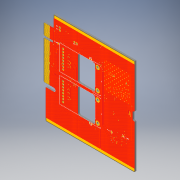
# Autodesk Inventor part: CardStandard
Saved by Autodesk Inventor 2018 (Build 220112000, 112)
## iProperties
Created: 2018-01-15
Part Number: CardStandard
Material: Epoxy Resin
Document SubType Name: Modeling
Designer: Bradley
Density: 1.14 g/cm^3
Appearance: Smooth - Medium Gray
Mass: 15.4834 g
Surface Area: 175.95 cm^2
Volume: 13.582 cm^3
Author: Bradley
Revision Number: 3.1
Autodesk Inventor part; units mm, degrees
ref_plane "YZ Plane" through (0, 0, 0) normal (1, 0, 0) x (0, 1, 0)
ref_plane "XZ Plane" through (0, 0, 0) normal (0, 1, 0) x (-1, 0, 0)
ref_plane "XY Plane" through (0, 0, 0) normal (0, 0, 1) x (1, 0, 0)
sketch "Sketch1" plane through (0, 0, 0) normal (0, 0, 1) x (1, 0, 0)
  line L0 (0, 36.15) -> (10, 36.15)
  line L1 (10, 36.15) -> (10, 47.9)
  line L2 (10, 47.9) -> (90.4, 47.9)
  line L3 (90.4, 47.9) -> (90.4, -47.9)
  line L4 (90.4, -47.9) -> (2, -47.9)
  line L5 (10, -15.15) -> (0, -15.15)
  line L6 (-5.5, 48) -> (90.5, 48) construction
  line L7 (90.5, 48) -> (90.5, -48) construction
  line L8 (90.5, -48) -> (-5.5, -48) construction
  line L9 (-5.5, -48) -> (-5.5, 48) construction
  line L10 (-5.4, 47.9) -> (-3.4, 47.9) construction
  line L11 (-3.4, 47.9) -> (-3.4, -47.9) construction
  line L12 (-3.4, -47.9) -> (-5.4, -47.9) construction
  line L13 (-5.4, -47.9) -> (-5.4, 47.9) construction
  line L14 (-3.4, 38.5) -> (7.85, 38.5) construction
  line L15 (7.85, 38.5) -> (7.85, -17.5) construction
  line L16 (7.85, -17.5) -> (-3.4, -17.5) construction
  line L17 (-3.4, -17.5) -> (-3.4, 38.5) construction
  line L18 (2, -47.9) -> (2, -18.65)
  line L19 (2, -18.65) -> (10, -18.65)
  arc A0 (10, -18.65) -> (10, -15.15) centre (10, -16.9) ccw
  line L20 (0, 24) -> (90.5, 24) construction
  circle A1 centre (-2.5, 47.1) radius 0.9 construction
  circle A2 centre (-0.7, 47.1) radius 0.9 construction
  circle A3 centre (1.1, 47.1) radius 0.9 construction
  circle A4 centre (2.9, 47.1) radius 0.9 construction
  circle A5 centre (4.7, 47.1) radius 0.9 construction
  circle A6 centre (6.5, 47.1) radius 0.9 construction
  circle A7 centre (8.3, 47.1) radius 0.9 construction
  circle A8 centre (-2.5, 45.3) radius 0.9 construction
  circle A9 centre (-0.7, 45.3) radius 0.9 construction
  circle A10 centre (1.1, 45.3) radius 0.9 construction
  circle A11 centre (2.9, 45.3) radius 0.9 construction
  circle A12 centre (4.7, 45.3) radius 0.9 construction
  circle A13 centre (6.5, 45.3) radius 0.9 construction
  circle A14 centre (8.3, 45.3) radius 0.9 construction
  circle A15 centre (-2.5, 43.5) radius 0.9 construction
  circle A16 centre (-0.7, 43.5) radius 0.9 construction
  circle A17 centre (1.1, 43.5) radius 0.9 construction
  circle A18 centre (2.9, 43.5) radius 0.9 construction
  circle A19 centre (4.7, 43.5) radius 0.9 construction
  circle A20 centre (6.5, 43.5) radius 0.9 construction
  circle A21 centre (8.3, 43.5) radius 0.9 construction
  circle A22 centre (-2.5, 41.7) radius 0.9 construction
  circle A23 centre (-0.7, 41.7) radius 0.9 construction
  circle A24 centre (1.1, 41.7) radius 0.9 construction
  circle A25 centre (2.9, 41.7) radius 0.9 construction
  circle A26 centre (4.7, 41.7) radius 0.9 construction
  circle A27 centre (6.5, 41.7) radius 0.9 construction
  circle A28 centre (8.3, 41.7) radius 0.9 construction
  circle A29 centre (-2.5, 39.9) radius 0.9 construction
  circle A30 centre (-0.7, 39.9) radius 0.9 construction
  circle A31 centre (1.1, 39.9) radius 0.9 construction
  circle A32 centre (2.9, 39.9) radius 0.9 construction
  circle A33 centre (4.7, 39.9) radius 0.9 construction
  circle A34 centre (6.5, 39.9) radius 0.9 construction
  circle A35 centre (8.3, 39.9) radius 0.9 construction
  line L21 (0, 36.15) -> (0, 24.95)
  line L22 (0, 24.95) -> (8.4, 24.95)
  arc A36 (8.4, 23.05) -> (8.4, 24.95) centre (8.4, 24) ccw
  line L23 (8.4, 23.05) -> (0, 23.05)
  line L24 (0, 23.05) -> (0, -15.15)
  point P0 (0, 0)
  point P1 (-5.5, 0)
  point P2 (90.4, 0)
  point P3 (90.5, 0)
  dimension "d0" = 51.3
  dimension "d1" = 95.8
  dimension "d3" = 10
  dimension "d20" = 96
  dimension "d21" = 96
  dimension "d22" = 0.1
  dimension "d23" = 0.1
  dimension "d24" = 2
  dimension "d25" = 0.1
  dimension "d28" = 11.25
  dimension "d29" = 56
  dimension "d31" = 9.5
  dimension "d32" = 30.5
  dimension "d34" = 3.5
  dimension "d35" = 12.15
  dimension "d36" = 39.15
  dimension "d37" = 14.5
  dimension "d38" = 1.15
  dimension "d39" = 1.8
  dimension "d42" = 1.8
  dimension "d45" = 1.8
  dimension "d48" = 2
  dimension "d49" = 3.4
  dimension "d50" = 1.9
  dimension "d51" = 8.4
  dimension "d52" = 24
  constraints: 50 end point, 37 centre point, 11 perpendicular, 7 parallel, 6 point on line, 6 tangent, 5 horizontal, 4 point on circle, 3 midpoint, 3 vertical, 2 collinear, 2 horizontal alignment, 68 other
  measures "d0" distance of L5.end L0.start
  measures "d1" distance of L2.end L3.end
  measures "d3" distance of L0.start L0.end
  measures "d20" distance of L6.start L6.end
  measures "d21" distance of L8.end L6.start
  measures "d22" distance between parallel lines of L2 L6
  measures "d23" distance between parallel lines of L7 L3
  measures "d24" distance between parallel lines of L13 L11
  measures "d25" distance between parallel lines of L13 L9
  measures "d28" distance of L15.end L16.end
  measures "d29" distance of L14.end L15.end
  measures "d31" distance between parallel lines of L14 L6
  measures "d32" distance between parallel lines of L8 L16
  measures "d34" distance between parallel lines of L5 L19
  measures "d35" distance between parallel lines of L20 L0
  measures "d36" distance between parallel lines of L5 L20
  measures "d37" distance between parallel lines of L20 L14
  measures "d38" distance between parallel lines of L19 L16
  measures "d39" diameter of A1
  measures "d42" distance of A1.centre A2.centre
  measures "d45" distance of A1.centre A8.centre
  measures "d48" distance between parallel lines of L18 L24
  measures "d49" distance between parallel lines of L24 L11
  measures "d50" distance between parallel lines of L23 L22
  measures "d51" distance of L21.end L22.end
  measures "d52" distance from line of point (0, 0) L20
extrude "Extrusion1" add sketch "Sketch1" along normal mid plane 1.6
chamfer "Chamfer1" distance 0.5 angle 45 4 edges at (0, 36.15, 0) (0, 24.95, 0) (0, 23.05, 0) (0, -15.15, 0)
fillet "Fillet1" radius 0.5 6 edges at (10, 36.15, 0) (10, 47.9, 0) (90.4, 47.9, 0) (90.4, -47.9, 0) (2, -47.9, 0) (2, -18.65, 0)
sketch "Sketch16" plane through (0, 0, 0.8) normal (0, 0, 1) x (1, 0, 0)
  arc A0 (2.5, -18.65) -> (2, -19.15) centre (2.5, -19.15) ccw projected
  line L0 (2, -19.15) -> (2, -47.4) projected
  arc A1 (2, -47.4) -> (2.5, -47.9) centre (2.5, -47.4) ccw projected
  line L1 (2.5, -47.9) -> (89.9, -47.9) projected
  arc A2 (89.9, -47.9) -> (90.4, -47.4) centre (89.9, -47.4) ccw projected
  line L2 (90.4, -47.4) -> (90.4, 47.4) projected
  arc A3 (90.4, 47.4) -> (89.9, 47.9) centre (89.9, 47.4) ccw projected
  line L3 (89.9, 47.9) -> (10.5, 47.9) projected
  arc A4 (10.5, 47.9) -> (10, 47.4) centre (10.5, 47.4) ccw projected
  line L4 (10, 47.4) -> (10, 36.65) projected
  arc A5 (9.5, 36.15) -> (10, 36.65) centre (9.5, 36.65) ccw projected
  line L5 (9.5, 36.15) -> (0.5, 36.15) projected
  line L6 (0, 35.65) -> (0.5, 36.15) projected
  line L7 (0, 35.65) -> (0, 25.45) projected
  line L8 (0.5, 24.95) -> (0, 25.45) projected
  line L9 (0.5, 24.95) -> (8.4, 24.95) projected
  arc A6 (8.4, 23.05) -> (8.4, 24.95) centre (8.4, 24) ccw projected
  line L10 (8.4, 23.05) -> (0.5, 23.05) projected
  line L11 (0, 22.55) -> (0.5, 23.05) projected
  line L12 (0, 22.55) -> (0, -14.65) projected
  line L13 (0.5, -15.15) -> (0, -14.65) projected
  line L14 (0.5, -15.15) -> (10, -15.15) projected
  arc A7 (10, -18.65) -> (10, -15.15) centre (10, -16.9) ccw projected
  line L15 (10, -18.65) -> (2.5, -18.65) projected
  line L16 (36.05, 26.5) -> (49.05, 26.5)
  line L17 (51.05, 24.5) -> (51.05, 3.5)
  line L18 (49.05, 1.5) -> (36.05, 1.5)
  line L19 (34.05, 3.5) -> (34.05, 24.5)
  line L20 (36.05, -1.5) -> (49.05, -1.5)
  line L21 (51.05, -3.5) -> (51.05, -24.5)
  line L22 (49.05, -26.5) -> (36.05, -26.5)
  line L23 (34.05, -24.5) -> (34.05, -3.5)
  line L24 (88.4, 3) -> (88.4, -3)
  arc A8 (88.4, -3) -> (89.4, -4) centre (89.4, -3) ccw
  arc A9 (90.4, -5) -> (89.4, -4) centre (89.4, -5) ccw
  arc A10 (89.4, 4) -> (88.4, 3) centre (89.4, 3) ccw
  line L25 (90.4, -47.4) -> (90.4, 47.4) projected
  arc A11 (89.4, 4) -> (90.4, 5) centre (89.4, 5) ccw
  arc A12 (36.05, 26.5) -> (34.05, 24.5) centre (36.05, 24.5) ccw
  arc A13 (51.05, 24.5) -> (49.05, 26.5) centre (49.05, 24.5) ccw
  arc A14 (49.05, 1.5) -> (51.05, 3.5) centre (49.05, 3.5) ccw
  arc A15 (51.05, -3.5) -> (49.05, -1.5) centre (49.05, -3.5) ccw
  arc A16 (49.05, -26.5) -> (51.05, -24.5) centre (49.05, -24.5) ccw
  arc A17 (34.05, -24.5) -> (36.05, -26.5) centre (36.05, -24.5) ccw
  arc A18 (36.05, -1.5) -> (34.05, -3.5) centre (36.05, -3.5) ccw
  arc A19 (34.05, 3.5) -> (36.05, 1.5) centre (36.05, 3.5) ccw
  point P0 (0, 0)
  point P1 (34.05, -1.5)
  point P2 (51.05, -26.5)
  point P3 (88.4, 0)
  dimension "d145" = 6
  dimension "d146" = 1
  dimension "d147" = 3
  dimension "d148" = 1.5
  dimension "d149" = 34.05
  dimension "d150" = 51.05
  dimension "d151" = 26.5
  dimension "d152" = 2
  constraints: 24 point on circle, 22 tangent, 18 end point, 12 centre point, 10 equal radius, 8 point on line, 4 parallel, 2 horizontal, 2 perpendicular, 1 collinear, 1 horizontal alignment, 1 midpoint, 1 vertical, 1 vertical alignment
  measures "d145" distance of L24.start L24.end
  measures "d146" radius of A11
  measures "d147" distance between parallel lines of L20 L18
  measures "d148" distance from line of point (0, 0) L18
  measures "d149" distance between parallel lines of L19 L12
  measures "d150" distance between parallel lines of L12 L17
  measures "d151" distance from line of point (0, 0) L22
  measures "d152" radius of A12
extrude "Extrusion6" cut sketch "Sketch16" against normal through all contours A9 A8 L24 A10 A11 L2 | L16 A13 L17 A14 L18 A19 L19 A12 | L20 A15 L21 A16 L22 A17 L23 A18
sketch "Sketch19" plane through (0, 0, 0.8) normal (0, 0, 1) x (1, 0, 0)
  line L0 (0, 22.55) -> (0, -14.65) projected
  line L1 (90.4, 5) -> (90.4, 47.4) projected
  line L2 (0, 47.8927) -> (90.4, 47.8927) construction
  line L3 (90.4, 47.8927) -> (90.4, -47.8927) construction
  line L4 (90.4, -47.8927) -> (0, -47.8927) construction
  line L5 (0, -47.8927) -> (0, 47.8927) construction
  point P0 (0, 0)
  constraints: 2 collinear, 1 midpoint, 2 other
decal "Decal4"
sketch "Sketch20" plane through (0, 0, -0.8) normal (0, 0, -1) x (-1, 0, 0)
  line L0 (-90.4, 47.4) -> (-90.4, 5) projected
  line L1 (0, -14.65) -> (0, 22.55) projected
  line L2 (-90.4, 47.8927) -> (0, 47.8927) construction
  line L3 (0, 47.8927) -> (0, -47.8927) construction
  line L4 (0, -47.8927) -> (-90.4, -47.8927) construction
  line L5 (-90.4, -47.8927) -> (-90.4, 47.8927) construction
  point P0 (0, 0)
  constraints: 2 collinear, 1 midpoint, 2 other
decal "Decal5"
sketch "Sketch21" plane through (0, 0, 0.8) normal (0, 0, 1) x (1, 0, 0)
  point P0 (0, 0)
  point P1 (53.55, -24)
  point P2 (53.55, -4)
  point P3 (53.55, 24)
  point P4 (53.55, 4)
  constraints: 4 other
hole "Hole9" at (53.55, -24, 0.8) at (53.55, -4, 0.8) at (53.55, 24, 0.8) at (53.55, 4, 0.8) direction (0, 0, -1) diameter 2.2 end through all
sketch "Sketch22" plane through (0, 0, 0.8) normal (0, 0, 1) x (1, 0, 0)
  point P0 (0, 0)
  point P1 (19.25, -17.81)
  point P2 (32.9, 34.25)
  point P3 (19.25, -12.73)
  point P4 (19.25, -10.19)
  point P5 (19.25, -7.65)
  point P6 (19.25, -5.11)
  point P7 (19.25, -15.27)
  point P8 (19.25, 20.35)
  point P9 (19.25, -20.35)
  point P10 (19.25, -22.89)
  point P11 (19.25, 17.81)
  point P12 (19.25, 15.27)
  point P13 (19.25, 22.89)
  point P14 (19.25, 12.73)
  point P15 (19.25, 10.19)
  point P16 (19.25, 7.65)
  point P17 (19.25, 5.11)
  point P18 (30.5, 34.25)
  point P19 (16, 39.5)
  point P20 (16, 37.05)
  constraints: 20 other
hole "Hole10" at (19.25, -17.81, 0.8) at (32.9, 34.25, 0.8) at (19.25, -12.73, 0.8) at (19.25, -10.19, 0.8) at (19.25, -7.65, 0.8) at (19.25, -5.11, 0.8) at (19.25, -15.27, 0.8) at (19.25, 20.35, 0.8) at (19.25, -20.35, 0.8) at (19.25, -22.89, 0.8) at (19.25, 17.81, 0.8) at (19.25, 15.27, 0.8) at (19.25, 22.89, 0.8) at (19.25, 12.73, 0.8) at (19.25, 10.19, 0.8) at (19.25, 7.65, 0.8) at (19.25, 5.11, 0.8) at (30.5, 34.25, 0.8) at (16, 39.5, 0.8) at (16, 37.05, 0.8) direction (0, 0, -1) diameter 1 end through all
sketch "Sketch23" plane through (0, 0, 0.8) normal (0, 0, 1) x (1, 0, 0)
  point P0 (0, 0)
  point P1 (82, 24.5)
  point P2 (69.5, 24.5)
  constraints: 2 other
hole "Hole11" at (82, 24.5, 0.8) at (69.5, 24.5, 0.8) direction (0, 0, -1) diameter 0.6 end through all
sketch "Sketch24" plane through (0, 0, 0.8) normal (0, 0, 1) x (1, 0, 0)
  point P0 (0, 0)
  point P1 (52.419, -22.869)
  point P2 (51.95, -24)
  point P3 (52.419, -25.131)
  point P4 (55.15, -24)
  point P5 (53.55, -5.6)
  point P6 (54.681, -5.131)
  point P7 (55.15, -4)
  point P8 (54.681, -2.869)
  point P9 (53.55, -2.4)
  point P10 (52.419, -2.869)
  point P11 (54.681, -22.869)
  point P12 (53.55, 22.4)
  point P13 (54.681, 22.869)
  point P14 (55.15, 24)
  point P15 (54.681, 25.131)
  point P16 (53.55, 25.6)
  point P17 (52.419, 25.131)
  point P18 (51.95, -4)
  point P19 (52.419, 22.869)
  point P20 (53.55, 2.4)
  point P21 (54.681, 2.869)
  point P22 (55.15, 4)
  point P23 (54.681, 5.131)
  point P24 (53.55, 5.6)
  point P25 (51.95, 24)
  point P26 (51.95, 4)
  point P27 (52.419, 2.869)
  point P28 (52.419, -5.131)
  point P29 (53.55, -25.6)
  point P30 (54.681, -25.131)
  point P31 (53.55, -22.4)
  point P32 (52.419, 5.131)
  constraints: 32 other
hole "Hole12" at (52.419, -22.869, 0.8) at (51.95, -24, 0.8) at (52.419, -25.131, 0.8) at (55.15, -24, 0.8) at (53.55, -5.6, 0.8) at (54.681, -5.131, 0.8) at (55.15, -4, 0.8) at (54.681, -2.869, 0.8) at (53.55, -2.4, 0.8) at (52.419, -2.869, 0.8) at (54.681, -22.869, 0.8) at (53.55, 22.4, 0.8) at (54.681, 22.869, 0.8) at (55.15, 24, 0.8) at (54.681, 25.131, 0.8) at (53.55, 25.6, 0.8) at (52.419, 25.131, 0.8) at (51.95, -4, 0.8) at (52.419, 22.869, 0.8) at (53.55, 2.4, 0.8) at (54.681, 2.869, 0.8) at (55.15, 4, 0.8) at (54.681, 5.131, 0.8) at (53.55, 5.6, 0.8) at (51.95, 24, 0.8) at (51.95, 4, 0.8) at (52.419, 2.869, 0.8) at (52.419, -5.131, 0.8) at (53.55, -25.6, 0.8) at (54.681, -25.131, 0.8) at (53.55, -22.4, 0.8) at (52.419, 5.131, 0.8) direction (0, 0, -1) diameter 0.35 end through all
sketch "Sketch25" plane through (0, 0, 0.8) normal (0, 0, 1) x (1, 0, 0)
  point P0 (0, 0)
  point P1 (80.65, 14.55)
  point P2 (79.45, 14.55)
  point P3 (79.15, 12.8)
  point P4 (79.1, 11.55)
  point P5 (77.3, 14.15)
  point P6 (76.1, 14.15)
  point P7 (77.25, 12.15)
  point P8 (77.25, 10.95)
  point P9 (74.55, 13)
  point P10 (72.7, 14.55)
  point P11 (69.6, 14.35)
  point P12 (69.8, 13)
  point P13 (69.8, 11.1)
  point P14 (72.3, 11.4)
  point P15 (66.9, 23.8)
  point P16 (68.5, 23.8)
  point P17 (64.9, 24.9)
  point P18 (68.5, 25.1)
  point P19 (66.9, 25.1)
  point P20 (64.9, 23.6)
  point P21 (82.7, 23.6)
  point P22 (81.3, 23.6)
  point P23 (82, 25.6)
  point P24 (82.7, 19.4)
  point P25 (81.3, 18.8)
  point P26 (83.8, 16.4)
  point P27 (85, 17)
  point P28 (85.05, 14.2)
  point P29 (81.1, 16.2)
  point P30 (77.95, 16.35)
  point P31 (75.05, 16.35)
  point P32 (71.85, 15.55)
  point P33 (66.5, 13.7)
  point P34 (65.6, 12.3)
  point P35 (70.6, 24.5)
  point P36 (84.5, 32)
  point P37 (76.5, 32)
  point P38 (68.5, 32)
  point P39 (72.5, 32)
  point P40 (80.5, 32)
  point P41 (64.5, 32)
  point P42 (82.5, 30)
  point P43 (74.5, 30)
  point P44 (66.5, 30)
  point P45 (70.5, 30)
  point P46 (78.5, 30)
  point P47 (62.5, 30)
  point P48 (84.5, 28)
  point P49 (76.5, 28)
  point P50 (68.5, 28)
  point P51 (72.5, 28)
  point P52 (80.5, 28)
  point P53 (64.5, 28)
  point P54 (74.5, 26)
  point P55 (66.5, 26)
  point P56 (70.5, 26)
  point P57 (78.5, 26)
  point P58 (62.5, 26)
  point P59 (84.5, 24)
  point P60 (76.5, 24)
  point P61 (72.5, 24)
  point P62 (74.5, 22)
  point P63 (66.5, 22)
  point P64 (70.5, 22)
  point P65 (78.5, 22)
  point P66 (62.5, 22)
  point P67 (84.5, 20)
  point P68 (76.5, 20)
  point P69 (68.5, 20)
  point P70 (72.5, 20)
  point P71 (80.5, 20)
  point P72 (64.5, 20)
  point P73 (74.5, 18)
  point P74 (66.5, 18)
  point P75 (70.5, 18)
  point P76 (78.5, 18)
  point P77 (62.5, 18)
  point P78 (84.5, 8)
  point P79 (76.5, 8)
  point P80 (68.5, 8)
  point P81 (72.5, 8)
  point P82 (80.5, 8)
  point P83 (64.5, 8)
  point P84 (82.5, 10)
  point P85 (74.5, 10)
  point P86 (66.5, 10)
  point P87 (70.5, 10)
  point P88 (78.5, 10)
  point P89 (62.5, 10)
  point P90 (82.5, 34)
  point P91 (74.5, 34)
  point P92 (66.5, 34)
  point P93 (70.5, 34)
  point P94 (56.2, 27.1)
  point P95 (62.5, 34)
  point P96 (60.5, 32)
  point P97 (60.5, 28)
  point P98 (60.5, 24)
  point P99 (60.5, 20)
  point P100 (60.5, 16)
  point P101 (62.5, 14)
  point P102 (60.5, 12)
  point P103 (64.5, 12)
  point P104 (64.5, 16)
  point P105 (13.5, 24.2)
  point P106 (15.3, 2.5)
  point P107 (15.3, -4.8)
  point P108 (55.3, -27)
  point P109 (73.075, -22.125)
  point P110 (77.7, -26.1)
  point P111 (25, 9.9)
  point P112 (25, 12.8)
  point P113 (25, 15.9)
  point P114 (24.59, 18.9)
  point P115 (24.6, -9.1)
  point P116 (25, -18.1)
  point P117 (25, -15.1)
  point P118 (25, -12.1)
  point P119 (80.4, -20.2)
  point P120 (80.4, -17.9)
  point P121 (62.6, 1.8)
  point P122 (60.2, 3.5)
  point P123 (25.25, 1.4)
  point P124 (25.25, -1.4)
  point P125 (28.5, 1.4)
  point P126 (13.8, 20)
  point P127 (67.5, -26.2)
  point P128 (58.86, 23)
  point P129 (67, -31)
  point P130 (72.9, -30.3)
  point P131 (69.3, -28.5)
  point P132 (67, -28.5)
  point P133 (55.5, 29.3)
  point P134 (57.7, 27.5)
  point P135 (57.7, 25.6)
  point P136 (72.5, -32.1)
  point P137 (87.6, 7.7)
  point P138 (70.3, -30.7)
  point P139 (68.7, -33.25)
  point P140 (70.432, -27.94)
  point P141 (77.1, -30.9)
  point P142 (72.3, -26.4)
  point P143 (58.3, 24.9)
  point P144 (67, -32.3)
  point P145 (72.4, -30.9)
  point P146 (69.3, -29.8)
  point P147 (51.75, -29.75)
  point P148 (70.001, -7.599)
  point P149 (69.209, -8.391)
  point P150 (77.45, -23.85)
  point P151 (6, -2.5)
  point P152 (30.5, -2.4)
  point P153 (26.4, 14.45)
  point P154 (6, -3.5)
  point P155 (31.1, -3)
  point P156 (29.9, -3)
  point P157 (29.9, -1.8)
  point P158 (26.4, 13.6)
  point P159 (6, -4.5)
  point P160 (31.7, -3.6)
  point P161 (29.3, -3.6)
  point P162 (29.3, -1.2)
  point P163 (26.4, 11.45)
  point P164 (58, 30.4)
  point P165 (17.6, 8.9)
  point P166 (26.4, 10.1)
  point P167 (9.8, 5.2)
  point P168 (20.7, -1.4)
  point P169 (24.5, -5.2)
  point P170 (6, 34.5)
  point P171 (6, 4.5)
  point P172 (6, 3.5)
  point P173 (27.596, 0.396)
  point P174 (26.804, -0.396)
  point P175 (25.3, 18.4)
  point P176 (25.8, 15.4)
  point P177 (25.8, 12.4)
  point P178 (25.3, -9.6)
  point P179 (25.8, -12.6)
  point P180 (25.8, -15.6)
  point P181 (6, 35.5)
  point P182 (25.2, 21)
  point P183 (26.4, -5.9)
  point P184 (32.4, -0.76)
  point P185 (70.6, 4.6)
  point P186 (70.75, 6.25)
  point P187 (6, 33.5)
  point P188 (6, 32.5)
  point P189 (6, 31.5)
  point P190 (6, 30.5)
  point P191 (6, 29.5)
  point P192 (6, 28.5)
  point P193 (6, 27.5)
  point P194 (6, 26.5)
  point P195 (6, 20.5)
  point P196 (6, 19.5)
  point P197 (6, 18.5)
  point P198 (6, 17.5)
  point P199 (6, 16.5)
  constraints: 244 other
hole "Hole13" at (80.65, 14.55, 0.8) at (79.45, 14.55, 0.8) at (79.15, 12.8, 0.8) at (79.1, 11.55, 0.8) at (77.3, 14.15, 0.8) at (76.1, 14.15, 0.8) at (77.25, 12.15, 0.8) at (77.25, 10.95, 0.8) at (74.55, 13, 0.8) at (72.7, 14.55, 0.8) at (69.6, 14.35, 0.8) at (69.8, 13, 0.8) at (69.8, 11.1, 0.8) at (72.3, 11.4, 0.8) at (66.9, 23.8, 0.8) at (68.5, 23.8, 0.8) at (64.9, 24.9, 0.8) at (68.5, 25.1, 0.8) at (66.9, 25.1, 0.8) at (64.9, 23.6, 0.8) at (82.7, 23.6, 0.8) at (81.3, 23.6, 0.8) at (82, 25.6, 0.8) at (82.7, 19.4, 0.8) at (81.3, 18.8, 0.8) at (83.8, 16.4, 0.8) at (85, 17, 0.8) at (85.05, 14.2, 0.8) at (81.1, 16.2, 0.8) at (77.95, 16.35, 0.8) at (75.05, 16.35, 0.8) at (71.85, 15.55, 0.8) at (66.5, 13.7, 0.8) at (65.6, 12.3, 0.8) at (70.6, 24.5, 0.8) at (84.5, 32, 0.8) at (76.5, 32, 0.8) at (68.5, 32, 0.8) at (72.5, 32, 0.8) at (80.5, 32, 0.8) at (64.5, 32, 0.8) at (82.5, 30, 0.8) at (74.5, 30, 0.8) at (66.5, 30, 0.8) at (70.5, 30, 0.8) at (78.5, 30, 0.8) at (62.5, 30, 0.8) at (84.5, 28, 0.8) at (76.5, 28, 0.8) at (68.5, 28, 0.8) direction (0, 0, -1) diameter 0.3 end through all and at (72.5, 28, 0.8) (80.5, 28, 0.8) (64.5, 28, 0.8) (74.5, 26, 0.8) (66.5, 26, 0.8) (70.5, 26, 0.8) (78.5, 26, 0.8) (62.5, 26, 0.8) (84.5, 24, 0.8) (76.5, 24, 0.8) (72.5, 24, 0.8) (74.5, 22, 0.8) (66.5, 22, 0.8) (70.5, 22, 0.8) (78.5, 22, 0.8) (62.5, 22, 0.8) (84.5, 20, 0.8) (76.5, 20, 0.8) (68.5, 20, 0.8) (72.5, 20, 0.8) (80.5, 20, 0.8) (64.5, 20, 0.8) (74.5, 18, 0.8) (66.5, 18, 0.8) (70.5, 18, 0.8) (78.5, 18, 0.8) (62.5, 18, 0.8) (84.5, 8, 0.8) (76.5, 8, 0.8) (68.5, 8, 0.8) (72.5, 8, 0.8) (80.5, 8, 0.8) (64.5, 8, 0.8) (82.5, 10, 0.8) (74.5, 10, 0.8) (66.5, 10, 0.8) (70.5, 10, 0.8) (78.5, 10, 0.8) (62.5, 10, 0.8) (82.5, 34, 0.8) (74.5, 34, 0.8) (66.5, 34, 0.8) (70.5, 34, 0.8) (56.2, 27.1, 0.8) (62.5, 34, 0.8) (60.5, 32, 0.8) (60.5, 28, 0.8) (60.5, 24, 0.8) (60.5, 20, 0.8) (60.5, 16, 0.8) (62.5, 14, 0.8) (60.5, 12, 0.8) (64.5, 12, 0.8) (64.5, 16, 0.8) (13.5, 24.2, 0.8) (15.3, 2.5, 0.8) (15.3, -4.8, 0.8) (55.3, -27, 0.8) (73.075, -22.125, 0.8) (77.7, -26.1, 0.8) (25, 9.9, 0.8) (25, 12.8, 0.8) (25, 15.9, 0.8) (24.59, 18.9, 0.8) (24.6, -9.1, 0.8) (25, -18.1, 0.8) (25, -15.1, 0.8) (25, -12.1, 0.8) (80.4, -20.2, 0.8) (80.4, -17.9, 0.8) (62.6, 1.8, 0.8) (60.2, 3.5, 0.8) (25.25, 1.4, 0.8) (25.25, -1.4, 0.8) (28.5, 1.4, 0.8) (13.8, 20, 0.8) (67.5, -26.2, 0.8) (58.86, 23, 0.8) (67, -31, 0.8) (72.9, -30.3, 0.8) (69.3, -28.5, 0.8) (67, -28.5, 0.8) (55.5, 29.3, 0.8) (57.7, 27.5, 0.8) (57.7, 25.6, 0.8) (72.5, -32.1, 0.8) (87.6, 7.7, 0.8) (70.3, -30.7, 0.8) (68.7, -33.25, 0.8) (70.432, -27.94, 0.8) (77.1, -30.9, 0.8) (72.3, -26.4, 0.8) (58.3, 24.9, 0.8) (67, -32.3, 0.8) (72.4, -30.9, 0.8) (69.3, -29.8, 0.8) (51.75, -29.75, 0.8) (70.001, -7.599, 0.8) (69.209, -8.391, 0.8) (77.45, -23.85, 0.8) (6, -2.5, 0.8) (30.5, -2.4, 0.8) (26.4, 14.45, 0.8) (6, -3.5, 0.8) (31.1, -3, 0.8) (29.9, -3, 0.8) (29.9, -1.8, 0.8) (26.4, 13.6, 0.8) (6, -4.5, 0.8) (31.7, -3.6, 0.8) (29.3, -3.6, 0.8) (29.3, -1.2, 0.8) (26.4, 11.45, 0.8) (58, 30.4, 0.8) (17.6, 8.9, 0.8) (26.4, 10.1, 0.8) (9.8, 5.2, 0.8) (20.7, -1.4, 0.8) (24.5, -5.2, 0.8) (6, 34.5, 0.8) (6, 4.5, 0.8) (6, 3.5, 0.8) (27.596, 0.396, 0.8) (26.804, -0.396, 0.8) (25.3, 18.4, 0.8) (25.8, 15.4, 0.8) (25.8, 12.4, 0.8) (25.3, -9.6, 0.8) (25.8, -12.6, 0.8) (25.8, -15.6, 0.8) (6, 35.5, 0.8) (25.2, 21, 0.8) (26.4, -5.9, 0.8) (32.4, -0.76, 0.8) (70.6, 4.6, 0.8) (70.75, 6.25, 0.8) (6, 33.5, 0.8) (6, 32.5, 0.8) (6, 31.5, 0.8) (6, 30.5, 0.8) (6, 29.5, 0.8) (6, 28.5, 0.8) (6, 27.5, 0.8) (6, 26.5, 0.8) (6, 20.5, 0.8) (6, 19.5, 0.8) (6, 18.5, 0.8) (6, 17.5, 0.8) (6, 16.5, 0.8) (6, 15.5, 0.8) (6, 14.5, 0.8) (60.7, 1.2, 0.8) (60.7, -1.2, 0.8) (6, 25.55, 0.8) (77.9, -27.6, 0.8) (82, -26.8, 0.8) (78.5, 34, 0.8) (74.4, -11, 0.8) (69.1, -6, 0.8) (17, 27.19, 0.8) (10.6, 25.9, 0.8) (6, 22.45, 0.8) (24.05, 9.7, 0.8) (24.05, 12.7, 0.8) (24.05, 15.7, 0.8) (24.05, 18.35, 0.8) (6, 21.5, 0.8) (24.05, -18.3, 0.8) (24.05, -15.3, 0.8) (24.05, -12.3, 0.8) (24.05, -9.65, 0.8) (8.8, 2.3, 0.8) (56.2, -44.3, 0.8) (56.6, 42.9, 0.8) (57.7, 44.4, 0.8) (24.2, 38.74, 0.8) (22, 39.4, 0.8) (6.2, 13.5, 0.8) (6.2, 12.5, 0.8) (6.2, 11.5, 0.8) (9.95, 22.05, 0.8) (12.35, 15.75, 0.8) (7.7, 2.3, 0.8) (10.8, 34.1, 0.8) (56.8, 28.2, 0.8) (19.95, 27.75, 0.8) (35.3, 28.2, 0.8) (48.3, -27.75, 0.8) (80, -24, 0.8) (82.6, -24, 0.8) (82.9, 14.75, 0.8) (81.05, 11.5, 0.8) (82.9, 13.25, 0.8) (26.4, -16.9, 0.8)
equation "\"d23\" = d22"
equation "\"d25\" = d22"
equation "\"d42\" = d39"
equation "\"d45\" = d39"
body "Solid1"
